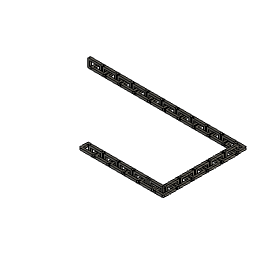
chain (Autodesk Fusion 360 design; units mm, degrees)
Autodesk Fusion 360 part; units mm, degrees
sketch "Sketch1" plane through (0, 0, 0) normal (0, 0, 1) x (1, 0, 0)
  line L0 (5, 2.5) -> (-5, 2.5)
  line L1 (-5, 2.5) -> (-5, -2.5)
  line L2 (-5, -2.5) -> (5, -2.5)
  line L3 (5, -2.5) -> (5, 2.5)
  line L4 (5, 2.5) -> (-5, -2.5) construction
  line L5 (-5, 2.5) -> (5, -2.5) construction
  line L6 (7, -4.5) -> (-7, -4.5)
  line L7 (-7, -4.5) -> (-7, 4.5)
  line L8 (-7, 4.5) -> (7, 4.5)
  line L9 (7, 4.5) -> (7, -4.5)
  line L10 (7, -4.5) -> (-7, 4.5) construction
  line L11 (-7, -4.5) -> (7, 4.5) construction
  dimension "d1" = 5
  dimension "d2" = 10
  dimension "d3" = 9
  dimension "d4" = 14
  constraint horizontal L0
  constraint perpendicular L0 L1
  constraint parallel L0 L2
  constraint parallel L1 L3
  constraint coincident L4 origin
  constraint coincident L5 origin
  constraint horizontal L6
  constraint perpendicular L6 L7
  constraint parallel L6 L8
  constraint parallel L7 L9
  constraint coincident L10 origin
  constraint coincident L11 origin
  measures "d1" distance of L0.end L1.end
  measures "d2" distance of L1.end L2.end
  measures "d3" distance of L6.end L7.end
  measures "d4" distance of L7.end L8.end
extrude "Extrude1" add sketch "Sketch1" along normal mid plane 2 makes body 1
fillet "Fillet1" radius 1 4 edges at (-7, -4.5, 0) (-7, 4.5, 0) (7, -4.5, 0) (7, 4.5, 0) on bodies 1
copy_body "Body->Comp1" bodies 1 removing the originals makes body 2 in component "Component"
pattern_linear "00000000-0000-0000-0000-000000000000" [suppressed]
component "Component" placed x (1, 0, 0) y (0, 1, 0) z (0, 0, 1) at (0, 0, 0)
component "Component" placed x (1, 0, 0) y (0, 0, 1) z (0, -1, 0) at (6, 0, 0)
component "Component" placed x (1, 0, 0) y (0, 1, 0) z (0, 0, 1) at (15, 0, 0)
component "Component" placed x (1, 0, 0) y (0, 0, 1) z (0, -1, 0) at (21, 0, 0)
component "Component" placed x (1, 0, 0) y (0, 1, 0) z (0, 0, 1) at (30, 0, 0)
component "Component" placed x (1, 0, 0) y (0, 0, 1) z (0, -1, 0) at (36, 0, 0)
component "Component" placed x (1, 0, 0) y (0, 1, 0) z (0, 0, 1) at (45, 0, 0)
component "Component" placed x (1, 0, 0) y (0, 0, 1) z (0, -1, 0) at (51, 0, 0)
component "Component" placed x (1, 0, 0) y (0, 1, 0) z (0, 0, 1) at (60, 0, 0)
component "Component" placed x (1, 0, 0) y (0, 0, 1) z (0, -1, 0) at (66, 0, 0)
component "Component" placed x (0, 1, 0) y (-1, 0, 0) z (0, 0, 1) at (72.4121, 2.8509, -1.7292)
component "Component" placed x (0, 1, 0) y (0, 0, 1) z (1, 0, 0) at (72.4121, 8.8509, -1.7292)
component "Component" placed x (0, 1, 0) y (-1, 0, 0) z (0, 0, 1) at (72.4121, 17.8509, -1.7292)
component "Component" placed x (0, 1, 0) y (0, 0, 1) z (1, 0, 0) at (72.4121, 23.8509, -1.7292)
component "Component" placed x (0, 1, 0) y (-1, 0, 0) z (0, 0, 1) at (72.4121, 32.8509, -1.7292)
component "Component" placed x (0, 1, 0) y (0, 0, 1) z (1, 0, 0) at (72.4121, 38.8509, -1.7292)
component "Component" placed x (0, 1, 0) y (-1, 0, 0) z (0, 0, 1) at (72.4121, 47.8509, -1.7292)
component "Component" placed x (0, 1, 0) y (0, 0, 1) z (1, 0, 0) at (72.4121, 53.8509, -1.7292)
component "Component" placed x (0, 1, 0) y (-1, 0, 0) z (0, 0, 1) at (72.4121, 62.8509, -1.7292)
component "Component" placed x (0, 1, 0) y (0, 0, 1) z (1, 0, 0) at (72.4121, 68.8509, -1.7292)
component "Component" placed x (0, 1, 0) y (-1, 0, 0) z (0, 0, 1) at (72.4121, 77.8509, -1.7292)
component "Component" placed x (0, 1, 0) y (0, 0, 1) z (1, 0, 0) at (72.4121, 83.8509, -1.7292)
component "Component" placed x (0, 1, 0) y (-1, 0, 0) z (0, 0, 1) at (72.4121, 92.8509, -1.7292)
component "Component" placed x (0, 1, 0) y (0, 0, 1) z (1, 0, 0) at (72.4121, 98.8509, -1.7292)
component "Component" placed x (0, 1, 0) y (-1, 0, 0) z (0, 0, 1) at (72.4121, 107.8509, -1.7292)
component "Component" placed x (0, 1, 0) y (0, 0, 1) z (1, 0, 0) at (72.4121, 113.8509, -1.7292)
component "Component" placed x (0, 1, 0) y (-1, 0, 0) z (0, 0, 1) at (72.4121, 122.8509, -1.7292)
component "Component" placed x (0, 1, 0) y (0, 0, 1) z (1, 0, 0) at (72.4121, 128.8509, -1.7292)
component "Component" placed x (0, 1, 0) y (-1, 0, 0) z (0, 0, 1) at (72.4121, 137.8509, -1.7292)
component "Component" placed x (0, 1, 0) y (0, 0, 1) z (1, 0, 0) at (72.4121, 143.8509, -1.7292)
component "Component" placed x (0, 1, 0) y (-1, 0, 0) z (0, 0, 1) at (72.4121, 152.8509, -1.7292)
component "Component" placed x (0, 1, 0) y (0, 0, 1) z (1, 0, 0) at (72.4121, 158.8509, -1.7292)
component "Component" placed x (0, 1, 0) y (-1, 0, 0) z (0, 0, 1) at (72.4121, 167.8509, -1.7292)
component "Component" placed x (0, 1, 0) y (0, 0, 1) z (1, 0, 0) at (72.4121, 173.8509, -1.7292)
component "Component" placed x (0, 1, 0) y (-1, 0, 0) z (0, 0, 1) at (72.4121, 182.8509, -1.7292)
component "Component" placed x (0, 1, 0) y (0, 0, 1) z (1, 0, 0) at (72.4121, 188.8509, -1.7292)
component "Component" placed x (0, 1, 0) y (-1, 0, 0) z (0, 0, 1) at (72.4121, 197.8509, -1.7292)
component "Component" placed x (0, 1, 0) y (0, 0, 1) z (1, 0, 0) at (72.4121, 203.8509, -1.7292)
component "Component" placed x (0, 1, 0) y (-1, 0, 0) z (0, 0, 1) at (72.4121, 212.8509, -1.7292)
component "Component" placed x (0, 1, 0) y (0, 0, 1) z (1, 0, 0) at (72.4121, 218.8509, -1.7292)
